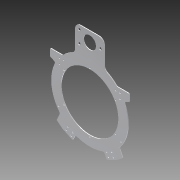
# Autodesk Inventor part: Tower_Top
Saved by Autodesk Inventor 2014 SP1 (Build 180222100, 222)
## iProperties
Created: 2012-02-04
Part Number: Tower_Top
Material: Aluminum-6061
Document SubType Name: Modeling
Designer: eagecat
Density: 2.71 g/cm^3
Mass: 552.559 g
Surface Area: 1384.69 cm^2
Volume: 203.896 cm^3
Appearance: Aluminum - Polished
Author: eagecat
Autodesk Inventor part; units mm, degrees
ref_plane "YZ Plane" through (0, 0, 0) normal (1, 0, 0) x (0, 1, 0)
ref_plane "XZ Plane" through (0, 0, 0) normal (0, 1, 0) x (-1, 0, 0)
ref_plane "XY Plane" through (0, 0, 0) normal (0, 0, 1) x (1, 0, 0)
sketch "Sketch1" plane through (0, 0, 0) normal (0, 0, 1) x (1, 0, 0)
  circle A0 centre (0, 0) radius 177.8
  circle A1 centre (0, 0) radius 132.461
  circle A2 centre (0, 0) radius 137.541 construction
  circle A3 centre (0, 137.541) radius 3.3782
  circle A4 centre (-119.114, 68.7705) radius 3.3782
  circle A5 centre (-119.114, -68.7705) radius 3.3782
  circle A6 centre (0, -137.541) radius 3.3782
  circle A7 centre (119.114, -68.7705) radius 3.3782
  circle A8 centre (119.114, 68.7705) radius 3.3782
  dimension "d2" = 275.082
  dimension "d0" = 355.6
  dimension "d1" = 264.922
  dimension "d3" = 6.7564
  dimension "d6" = 360
  constraints: 8 centre point, 3 coincident, 1 vertical alignment, 15 other
  measures "d0" diameter of A0
  measures "d1" diameter of A1
  measures "d3" diameter of A3
extrude "Extrusion1" add sketch "Sketch1" along normal blind 3.175
sketch "Sketch2" plane through (0, 0, 0) normal (0, 0, 1) x (1, 0, 0)
  line L0 (177.8, 120.269) -> (152.4, 120.269) construction
  line L1 (152.4, 120.269) -> (152.4, 94.869) construction
  line L2 (152.4, 94.869) -> (177.8, 94.869) construction
  line L3 (177.8, 94.869) -> (177.8, 120.269) construction
  line L4 (-176.2125, 96.4565) -> (-176.2125, 118.6815) construction
  line L5 (-176.2125, 118.6815) -> (-153.9875, 118.6815) construction
  line L6 (-153.9875, 118.6815) -> (-153.9875, 96.4565) construction
  line L7 (-153.9875, 96.4565) -> (-176.2125, 96.4565) construction
  line L8 (-177.8, 120.269) -> (-152.4, 120.269) construction
  line L9 (-177.8, 94.869) -> (-177.8, 120.269) construction
  line L10 (-152.4, 94.869) -> (-177.8, 94.869) construction
  line L11 (-152.4, 120.269) -> (-152.4, 94.869) construction
  line L12 (-131.8407, -121.2351) -> (-142.3056, -143.6999) construction
  line L13 (-111.6944, -130.6201) -> (-131.8407, -121.2351) construction
  line L14 (-122.1593, -153.0849) -> (-111.6944, -130.6201) construction
  line L15 (-142.3056, -143.6999) -> (-122.1593, -153.0849) construction
  line L16 (-144.4922, -144.6342) -> (-132.5322, -118.9602) construction
  line L17 (-121.4678, -155.3598) -> (-144.4922, -144.6342) construction
  line L18 (-109.5078, -129.6858) -> (-121.4678, -155.3598) construction
  line L19 (-132.5322, -118.9602) -> (-109.5078, -129.6858) construction
  line L20 (-108.1537, -135.5008) -> (-124.2421, -170.0373) construction
  line L21 (-81.532, -189.9334) -> (-124.2421, -170.0373) construction
  line L22 (-63.9062, -159.6156) -> (-77.3132, -188.396) construction
  line L23 (-108.1537, -135.5008) -> (-65.4435, -155.3968) construction
  circle A0 centre (109.1684, -166.5516) radius 3.3782 construction
  circle A1 centre (86.144, -177.2772) radius 3.3782 construction
  circle A2 centre (101.1241, -149.2833) radius 3.3782 construction
  circle A3 centre (78.0998, -160.0089) radius 3.3782 construction
  line L24 (108.1537, -135.5009) -> (124.2422, -170.0374) construction
  line L25 (108.1537, -135.5009) -> (62.5655, -156.7376) construction
  line L26 (62.5655, -156.7376) -> (78.6539, -191.2742) construction
  line L27 (78.6539, -191.2742) -> (124.2422, -170.0374) construction
  line L28 (142.3056, -143.6999) -> (131.8407, -121.2351) construction
  line L29 (122.1593, -153.0849) -> (142.3056, -143.6999) construction
  line L30 (111.6944, -130.6201) -> (122.1593, -153.0849) construction
  line L31 (131.8407, -121.2351) -> (111.6944, -130.6201) construction
  line L32 (132.5322, -118.9602) -> (144.4922, -144.6342) construction
  line L33 (109.5078, -129.6858) -> (132.5322, -118.9602) construction
  line L34 (121.4678, -155.3598) -> (109.5078, -129.6858) construction
  line L35 (144.4922, -144.6342) -> (121.4678, -155.3598) construction
  line L36 (0, 251.6148) -> (0, -265.089) construction
  line L37 (-256.032, 0) -> (256.032, 0) construction
  circle A4 centre (0, 0) radius 132.461 construction
  circle A5 centre (119.114, 68.7705) radius 3.3782 construction
  circle A6 centre (119.114, -68.7705) radius 3.3782 construction
  circle A7 centre (0, -137.541) radius 3.3782 construction
  circle A8 centre (-119.114, -68.7705) radius 3.3782 construction
  circle A9 centre (-119.114, 68.7705) radius 3.3782 construction
  circle A10 centre (0, 137.541) radius 3.3782 construction
  circle A11 centre (0, 0) radius 177.8 construction
  line L38 (-152.9297, -147.7089) -> (-124.2421, -170.0373)
  line L39 (-78.6539, -191.2741) -> (-124.2421, -170.0373)
  arc A12 (-58.5237, -167.8923) -> (-70.1072, -172.927) centre (-61.473, -176.9492) ccw
  line L40 (-70.1072, -172.927) -> (-78.6539, -191.2741)
  arc A13 (-138.5859, -111.3858) -> (-58.5237, -167.8923) centre (0, 0) ccw
  line L41 (-152.9297, -147.7089) -> (-139.107, -118.0362)
  arc A14 (-139.107, -118.0362) -> (-138.5859, -111.3858) centre (-147.7411, -114.0141) ccw
  line L42 (131.8407, -121.2351) -> (142.3056, -143.6999) construction
  line L43 (111.6944, -130.6201) -> (131.8407, -121.2351) construction
  line L44 (122.1593, -153.0849) -> (111.6944, -130.6201) construction
  line L45 (142.3056, -143.6999) -> (122.1593, -153.0849) construction
  line L46 (144.4922, -144.6342) -> (132.5322, -118.9602) construction
  line L47 (121.4678, -155.3598) -> (144.4922, -144.6342) construction
  line L48 (109.5078, -129.6858) -> (121.4678, -155.3598) construction
  line L49 (132.5322, -118.9602) -> (109.5078, -129.6858) construction
  circle A15 centre (109.1684, -166.5516) radius 3.3782 construction
  circle A16 centre (86.144, -177.2772) radius 3.3782 construction
  circle A17 centre (101.1241, -149.2833) radius 3.3782 construction
  circle A18 centre (78.0998, -160.0089) radius 3.3782 construction
  line L50 (108.1537, -135.5009) -> (124.2422, -170.0374) construction
  line L51 (78.6539, -191.2742) -> (124.2422, -170.0374) construction
  line L52 (62.5655, -156.7376) -> (78.6539, -191.2742) construction
  line L53 (108.1537, -135.5009) -> (62.5655, -156.7376) construction
  line L54 (152.9297, -147.7089) -> (124.2422, -170.0374)
  line L55 (78.6539, -191.2742) -> (124.2422, -170.0374)
  arc A19 (70.1072, -172.927) -> (58.5237, -167.8923) centre (61.473, -176.9492) ccw
  line L56 (70.1072, -172.927) -> (78.6539, -191.2742)
  arc A20 (58.5237, -167.8923) -> (138.5859, -111.3858) centre (0, 0) ccw
  line L57 (152.9297, -147.7089) -> (139.107, -118.0362)
  arc A21 (138.5859, -111.3858) -> (139.107, -118.0362) centre (147.7411, -114.0141) ccw
  line L58 (-182.88, 91.694) -> (-164.4375, 83.1028)
  line L59 (-182.88, 125.349) -> (-128.7113, 125.349)
  line L60 (-182.88, 125.349) -> (-182.88, 91.694)
  arc A22 (-161.3561, 74.6795) -> (-164.4375, 83.1028) centre (-167.1189, 77.3467) ccw
  arc A23 (-128.7113, 125.349) -> (-124.273, 127.1577) centre (-128.7113, 131.699) ccw
  arc A24 (-124.273, 127.1577) -> (-161.3561, 74.6795) centre (0, 0) ccw
  line L61 (176.2125, 96.4565) -> (176.2125, 118.6815) construction
  line L62 (176.2125, 118.6815) -> (153.9875, 118.6815) construction
  line L63 (153.9875, 118.6815) -> (153.9875, 96.4565) construction
  line L64 (153.9875, 96.4565) -> (176.2125, 96.4565) construction
  line L65 (177.8, 120.269) -> (152.4, 120.269) construction
  line L66 (177.8, 94.869) -> (177.8, 120.269) construction
  line L67 (152.4, 94.869) -> (177.8, 94.869) construction
  line L68 (152.4, 120.269) -> (152.4, 94.869) construction
  circle A25 centre (119.114, 68.7705) radius 3.3782 construction
  line L69 (182.88, 91.694) -> (164.4375, 83.1028)
  line L70 (182.88, 125.349) -> (128.7113, 125.349)
  line L71 (182.88, 125.349) -> (182.88, 91.694)
  arc A26 (164.4375, 83.1028) -> (161.3561, 74.6795) centre (167.1189, 77.3467) ccw
  arc A27 (124.273, 127.1577) -> (128.7113, 125.349) centre (128.7113, 131.699) ccw
  arc A28 (161.3561, 74.6795) -> (124.273, 127.1577) centre (0, 0) ccw
  arc A29 (-108.9915, -163.1779) -> (-109.3417, -163.1777) centre (-109.1683, -166.5515) ccw projected
  arc A30 (-85.9671, -173.9036) -> (-86.3174, -173.9034) centre (-86.144, -177.2771) ccw projected
  arc A31 (-100.9473, -145.9097) -> (-101.2975, -145.9095) centre (-101.1241, -149.2832) ccw projected
  arc A32 (-77.9229, -156.6353) -> (-78.2732, -156.6351) centre (-78.0998, -160.0089) ccw projected
  line L72 (-83.178, -156.6326) -> (-78.2732, -156.6351) projected
  line L73 (-77.9229, -156.6353) -> (-73.2656, -156.6377) projected
  arc A33 (-73.0184, -163.3851) -> (-73.2656, -156.6377) centre (-73.0198, -160.0069) ccw projected
  line L74 (-73.0184, -163.3851) -> (-83.1784, -163.389) projected
  arc A34 (-83.178, -156.6326) -> (-83.1784, -163.389) centre (-83.1797, -160.0108) ccw projected
  line L75 (-114.2466, -163.1752) -> (-109.3417, -163.1777) projected
  line L76 (-108.9915, -163.1779) -> (-104.3342, -163.1803) projected
  arc A35 (-104.087, -169.9277) -> (-104.3342, -163.1803) centre (-104.0883, -166.5495) ccw projected
  line L77 (-104.087, -169.9277) -> (-114.247, -169.9316) projected
  arc A36 (-114.2466, -163.1752) -> (-114.247, -169.9316) centre (-114.2483, -166.5534) ccw projected
  line L78 (-106.2024, -145.907) -> (-101.2975, -145.9095) projected
  line L79 (-100.9473, -145.9097) -> (-96.29, -145.912) projected
  arc A37 (-96.0428, -152.6595) -> (-96.29, -145.912) centre (-96.0441, -149.2813) ccw projected
  line L80 (-96.0428, -152.6595) -> (-106.2028, -152.6634) projected
  arc A38 (-106.2024, -145.907) -> (-106.2028, -152.6634) centre (-106.2041, -149.2852) ccw projected
  line L81 (-85.9671, -173.9036) -> (-81.3098, -173.9059) projected
  arc A39 (-81.0627, -180.6534) -> (-81.3098, -173.9059) centre (-81.064, -177.2752) ccw projected
  line L82 (-81.0627, -180.6534) -> (-91.2227, -180.6573) projected
  arc A40 (-91.2223, -173.9009) -> (-91.2227, -180.6573) centre (-91.224, -177.2791) ccw projected
  line L83 (-91.2223, -173.9009) -> (-86.3174, -173.9034) projected
  arc A41 (-63.9062, -159.6156) -> (-65.4435, -155.3968) centre (-66.7842, -158.2749) ccw projected
  arc A42 (-81.532, -189.9334) -> (-77.3132, -188.396) centre (-80.1912, -187.0553) ccw projected
  dimension "d11" = 6.35
  dimension "d12" = 9.525
  dimension "d13" = 9.525
  dimension "d14" = 6.35
  dimension "d23" = 3.175
  dimension "d24" = 5.08
  dimension "d25" = 5.08
  dimension "d26" = 6.35
  dimension "d27" = 6.35
  constraints: 36 end point, 28 point on circle, 20 symmetric about line, 17 centre point, 8 tangent, 3 perpendicular, 2 concentric, 2 parallel, 2 point on line, 1 collinear, 11 other
  measures "d11" distance from line of L17 L38.start
  measures "d12" radius of A12
  measures "d13" radius of A14
  measures "d14" distance between parallel lines of L16 L41
  measures "d23" distance from line of L10 L58.start
  measures "d24" distance between parallel lines of L60 L9
  measures "d25" distance between parallel lines of L59 L8
  measures "d26" radius of A23
  measures "d27" radius of A22
extrude "Extrusion5" add sketch "Sketch2" along normal blind 3.175 contours L41 A14 A13 L78 A38 L80 A37 A34 L74 A33 A12 L40 A42 L39 L38 | A42 L40 L39 | A13 A37 L80 A38 L78 | A13 A33 L74 A34 | L54 L55 L56 A19 A20 A21 L57 | L60 L59 A23 A24 A22 L58 | L69 A26 A28 A27 L70 L71 | L76 A35 L77 A36 L75 A29 | L81 A39 L82 A40 L83 A30
sketch "Sketch3" plane through (0, 0, 0) normal (0, 0, 1) x (1, 0, 0)
  circle A0 centre (109.1684, -166.5516) radius 3.3782 construction
  circle A1 centre (86.144, -177.2772) radius 3.3782 construction
  circle A2 centre (101.1241, -149.2833) radius 3.3782 construction
  circle A3 centre (78.0998, -160.0089) radius 3.3782 construction
  line L0 (124.2422, -170.0374) -> (108.1537, -135.5009) construction
  line L1 (124.2422, -170.0374) -> (78.6539, -191.2742) construction
  line L2 (78.6539, -191.2742) -> (62.5655, -156.7376) construction
  line L3 (62.5655, -156.7376) -> (108.1537, -135.5009) construction
  line L4 (-124.2421, -170.0373) -> (-108.1537, -135.5008) construction
  line L5 (-65.4435, -155.3968) -> (-108.1537, -135.5008) construction
  line L6 (-77.3132, -188.396) -> (-63.9062, -159.6156) construction
  line L7 (-124.2421, -170.0373) -> (-81.532, -189.9334) construction
  circle A4 centre (-109.1684, -166.5516) radius 3.3782
  circle A5 centre (-86.144, -177.2772) radius 3.3782
  circle A6 centre (-78.0998, -160.0089) radius 3.3782
  circle A7 centre (-101.1241, -149.2833) radius 3.3782
  circle A8 centre (78.0998, -160.0089) radius 3.3782
  circle A9 centre (86.144, -177.2772) radius 3.3782
  circle A10 centre (109.1684, -166.5516) radius 3.3782
  circle A11 centre (101.1241, -149.2833) radius 3.3782
  arc A12 (-108.9915, -163.1779) -> (-109.3417, -163.1777) centre (-109.1683, -166.5515) ccw projected
  arc A13 (-85.9671, -173.9036) -> (-86.3174, -173.9034) centre (-86.144, -177.2771) ccw projected
  arc A14 (-100.9473, -145.9097) -> (-101.2975, -145.9095) centre (-101.1241, -149.2832) ccw projected
  arc A15 (-77.9229, -156.6353) -> (-78.2732, -156.6351) centre (-78.0998, -160.0089) ccw projected
  line L8 (-86.3174, -173.9034) -> (-91.2223, -173.9009) projected
  arc A16 (-91.2223, -173.9009) -> (-91.2227, -180.6573) centre (-91.224, -177.2791) ccw projected
  line L9 (-91.2227, -180.6573) -> (-81.0627, -180.6534) projected
  arc A17 (-81.0627, -180.6534) -> (-81.3098, -173.9059) centre (-81.064, -177.2752) ccw projected
  line L10 (-81.3098, -173.9059) -> (-85.9671, -173.9036) projected
  line L11 (-101.2975, -145.9095) -> (-106.2024, -145.907) projected
  arc A18 (-106.2024, -145.907) -> (-106.2028, -152.6634) centre (-106.2041, -149.2852) ccw projected
  line L12 (-106.2028, -152.6634) -> (-96.0428, -152.6595) projected
  arc A19 (-96.0428, -152.6595) -> (-96.29, -145.912) centre (-96.0441, -149.2813) ccw projected
  line L13 (-96.29, -145.912) -> (-100.9473, -145.9097) projected
  line L14 (-109.3417, -163.1777) -> (-114.2466, -163.1752) projected
  arc A20 (-114.2466, -163.1752) -> (-114.247, -169.9316) centre (-114.2483, -166.5534) ccw projected
  line L15 (-114.247, -169.9316) -> (-104.087, -169.9277) projected
  arc A21 (-104.087, -169.9277) -> (-104.3342, -163.1803) centre (-104.0883, -166.5495) ccw projected
  line L16 (-104.3342, -163.1803) -> (-108.9915, -163.1779) projected
  line L17 (-78.2732, -156.6351) -> (-83.178, -156.6326) projected
  arc A22 (-83.178, -156.6326) -> (-83.1784, -163.389) centre (-83.1797, -160.0108) ccw projected
  line L18 (-83.1784, -163.389) -> (-73.0184, -163.3851) projected
  arc A23 (-73.0184, -163.3851) -> (-73.2656, -156.6377) centre (-73.0198, -160.0069) ccw projected
  line L19 (-73.2656, -156.6377) -> (-77.9229, -156.6353) projected
  arc A24 (-63.9062, -159.6156) -> (-65.4435, -155.3968) centre (-66.7842, -158.2749) ccw projected
  arc A25 (-81.532, -189.9334) -> (-77.3132, -188.396) centre (-80.1912, -187.0553) ccw projected
  point P0 (0, 0)
  constraints: 8 centre point, 8 equal radius, 4 coincident
extrude "Extrusion4" cut sketch "Sketch3" along normal blind 127 contours A4 | A5 | A6 | A7 | A8 | A9 | A10 | A11
fillet "Fillet1" radius 3.175 1 edges at (-182.88, 125.349, 1.5875)
fillet "Fillet2" radius 3.175 1 edges at (-182.88, 91.694, 1.5875)
fillet "Fillet3" radius 3.175 8 edges at (182.88, 125.349, 1.5875) (182.88, 91.694, 1.5875) (152.9297, -147.7089, 1.5875) (124.2422, -170.0374, 1.5875) (78.6539, -191.2742, 1.5875) (-78.6539, -191.2741, 1.5875) (-124.2421, -170.0373, 1.5875) (-152.9297, -147.7089, 1.5875)
sketch "Sketch4" plane through (0, 0, 0) normal (0, 0, -1) x (-1, 0, 0)
  arc A0 (130.175, 72.644) -> (133.35, 69.469) centre (133.35, 72.644) ccw construction
  line L0 (146.05, 69.469) -> (133.35, 69.469) construction
  arc A1 (146.05, 69.469) -> (149.225, 72.644) centre (146.05, 72.644) ccw construction
  line L1 (149.225, 85.344) -> (149.225, 72.644) construction
  line L2 (149.225, 85.344) -> (147.1295, 85.344) construction
  line L3 (147.1295, 85.344) -> (147.1295, 88.519) construction
  line L4 (147.1295, 88.519) -> (148.717, 88.519) construction
  line L5 (148.717, 88.519) -> (148.717, 120.269) construction
  line L6 (114.3, 120.269) -> (148.717, 120.269) construction
  arc A2 (114.3, 120.269) -> (111.125, 117.094) centre (114.3, 117.094) ccw construction
  line L7 (111.125, 98.044) -> (111.125, 117.094) construction
  arc A3 (111.125, 98.044) -> (114.3, 94.869) centre (114.3, 98.044) ccw construction
  line L8 (114.3, 94.869) -> (127, 94.869) construction
  arc A4 (130.175, 91.694) -> (127, 94.869) centre (127, 91.694) ccw construction
  line L9 (130.175, 91.694) -> (130.175, 72.644) construction
  arc A5 (136.3218, 77.089) -> (143.0782, 77.089) centre (139.7, 77.089) ccw construction
  line L10 (136.3218, 77.089) -> (136.3218, 87.249) construction
  arc A6 (143.0782, 87.249) -> (136.3218, 87.249) centre (139.7, 87.249) ccw construction
  line L11 (143.0782, 87.249) -> (143.0782, 77.089) construction
  line L12 (143.0782, 112.649) -> (143.0782, 102.489) construction
  arc A7 (136.3218, 102.489) -> (143.0782, 102.489) centre (139.7, 102.489) ccw construction
  line L13 (136.3218, 102.489) -> (136.3218, 112.649) construction
  arc A8 (143.0782, 112.649) -> (136.3218, 112.649) centre (139.7, 112.649) ccw construction
  line L14 (124.0282, 112.649) -> (124.0282, 102.489) construction
  arc A9 (117.2718, 102.489) -> (124.0282, 102.489) centre (120.65, 102.489) ccw construction
  line L15 (117.2718, 102.489) -> (117.2718, 112.649) construction
  arc A10 (124.0282, 112.649) -> (117.2718, 112.649) centre (120.65, 112.649) ccw construction
  arc A11 (-133.35, 69.469) -> (-130.175, 72.644) centre (-133.35, 72.644) ccw construction
  line L16 (-130.175, 91.694) -> (-130.175, 72.644) construction
  arc A12 (-127, 94.869) -> (-130.175, 91.694) centre (-127, 91.694) ccw construction
  line L17 (-114.3, 94.869) -> (-127, 94.869) construction
  arc A13 (-114.3, 94.869) -> (-111.125, 98.044) centre (-114.3, 98.044) ccw construction
  line L18 (-111.125, 98.044) -> (-111.125, 117.094) construction
  arc A14 (-111.125, 117.094) -> (-114.3, 120.269) centre (-114.3, 117.094) ccw construction
  line L19 (-114.3, 120.269) -> (-148.717, 120.269) construction
  line L20 (-148.717, 88.519) -> (-148.717, 120.269) construction
  line L21 (-147.1295, 88.519) -> (-148.717, 88.519) construction
  line L22 (-147.1295, 85.344) -> (-147.1295, 88.519) construction
  line L23 (-149.225, 85.344) -> (-147.1295, 85.344) construction
  line L24 (-149.225, 85.344) -> (-149.225, 72.644) construction
  arc A15 (-149.225, 72.644) -> (-146.05, 69.469) centre (-146.05, 72.644) ccw construction
  line L25 (-146.05, 69.469) -> (-133.35, 69.469) construction
  arc A16 (-143.0782, 77.089) -> (-136.3218, 77.089) centre (-139.7, 77.089) ccw construction
  line L26 (-143.0782, 87.249) -> (-143.0782, 77.089) construction
  arc A17 (-136.3218, 87.249) -> (-143.0782, 87.249) centre (-139.7, 87.249) ccw construction
  line L27 (-136.3218, 77.089) -> (-136.3218, 87.249) construction
  line L28 (-143.0782, 112.649) -> (-143.0782, 102.489) construction
  arc A18 (-136.3218, 112.649) -> (-143.0782, 112.649) centre (-139.7, 112.649) ccw construction
  line L29 (-136.3218, 102.489) -> (-136.3218, 112.649) construction
  arc A19 (-143.0782, 102.489) -> (-136.3218, 102.489) centre (-139.7, 102.489) ccw construction
  line L30 (-124.0282, 112.649) -> (-124.0282, 102.489) construction
  arc A20 (-117.2718, 112.649) -> (-124.0282, 112.649) centre (-120.65, 112.649) ccw construction
  line L31 (-117.2718, 102.489) -> (-117.2718, 112.649) construction
  arc A21 (-124.0282, 102.489) -> (-117.2718, 102.489) centre (-120.65, 102.489) ccw construction
  line L32 (120.65, 112.649) -> (120.65, 102.489) construction
  line L33 (139.7, 112.649) -> (139.7, 102.489) construction
  line L34 (139.7, 87.249) -> (139.7, 77.089) construction
  circle A22 centre (120.65, 107.569) radius 3.3782
  circle A23 centre (139.7, 107.569) radius 3.3782
  circle A24 centre (139.7, 82.169) radius 3.3782
  line L35 (-139.7, 112.649) -> (-139.7, 102.489) construction
  line L36 (-120.65, 112.649) -> (-120.65, 102.489) construction
  line L37 (-139.7, 87.249) -> (-139.7, 77.089) construction
  circle A25 centre (-139.7, 107.569) radius 3.3782
  circle A26 centre (-120.65, 107.569) radius 3.3782
  circle A27 centre (-139.7, 82.169) radius 3.3782
  constraints: 12 end point, 6 centre point, 6 equal length, 6 midpoint, 4 tangent
extrude "Extrusion6" cut sketch "Sketch4" against normal blind 25.4
sketch "Sketch6" plane through (0, 0, 3.175) normal (0, 0, 1) x (1, 0, 0)
  arc A0 (138.5859, -111.3858) -> (161.3561, 74.6795) centre (0, 0) ccw construction
  arc A1 (138.5859, -111.3858) -> (161.3561, 74.6795) centre (0, 0) ccw construction
  circle A2 centre (-48.7258, 267.14) radius 2.5 construction
  circle A3 centre (-48.7258, 267.14) radius 5.95 construction
  circle A4 centre (48.7258, 238.76) radius 2.5 construction
  circle A5 centre (48.7258, 238.76) radius 5.95 construction
  circle A6 centre (-48.7258, 210.38) radius 2.5 construction
  circle A7 centre (-48.7258, 210.38) radius 5.95 construction
  circle A8 centre (48.7258, 238.76) radius 7.1 construction
  circle A9 centre (-48.7258, 267.14) radius 7.1 construction
  circle A10 centre (-48.7258, 210.38) radius 7.1 construction
  line L0 (-42.3758, 286.19) -> (42.3758, 286.19)
  arc A11 (-42.3758, 286.19) -> (-67.7758, 260.79) centre (-42.3758, 260.79) ccw
  arc A12 (67.7758, 260.79) -> (42.3758, 286.19) centre (42.3758, 260.79) ccw
  line L1 (-67.7758, 260.79) -> (-67.7758, 180.5783)
  line L2 (67.7758, 260.79) -> (67.7758, 180.5783)
  arc A13 (-81.5289, 158.006) -> (-67.7758, 180.5783) centre (-93.1758, 180.5783) ccw
  arc A14 (67.7758, 180.5783) -> (81.5289, 158.006) centre (93.1758, 180.5783) ccw
  circle A15 centre (-48.7258, 267.14) radius 6.223
  circle A16 centre (48.7258, 238.76) radius 6.223
  circle A17 centre (-48.7258, 210.38) radius 6.223
  arc A18 (81.5289, 158.006) -> (-81.5289, 158.006) centre (0, 0) ccw
  circle A19 centre (0, 238.76) radius 29.21
  point P0 (124.273, 127.1577)
  point P1 (25.4, 175.9764)
  point P2 (-25.4, 175.9764)
  point P3 (-124.273, 127.1577)
  dimension "d50" = 25.4
  dimension "d51" = 25.4
  dimension "d52" = 19.05
  dimension "d53" = 19.05
  dimension "d54" = 19.05
  dimension "d55" = 25.4
  dimension "d56" = 12.446
  dimension "d57" = 12.446
  dimension "d58" = 12.446
  dimension "d63" = 58.42
  constraints: 12 point on circle, 9 centre point, 8 tangent, 6 end point, 4 coincident, 2 equal radius, 1 horizontal, 1 parallel, 1 perpendicular, 1 other
  measures "d50" radius of A11
  measures "d51" radius of A13
  measures "d52" distance from line of L1 A3.centre
  measures "d53" distance from line of L0 A2.centre
  measures "d54" distance from line of L2 A8.centre
  measures "d55" radius of A14
  measures "d56" diameter of A15
  measures "d57" diameter of A16
  measures "d58" diameter of A17
  measures "d63" diameter of A19
extrude "Extrusion10" add sketch "Sketch6" against normal blind 3.175
sketch "Sketch7" plane through (0, 0, 0) normal (0, 0, -1) x (-1, 0, 0)
  circle A0 centre (-143.8474, -86.121) radius 3.3782 projected
  circle A1 centre (143.8474, -86.121) radius 3.3782 projected
  point P0 (245.6114, -73.0705)
  constraints: 1 other
extrude "Extrusion11" cut sketch "Sketch7" against normal blind 25.4
equation "\"d57\" = d56"
equation "\"d58\" = d56"
body "Solid1"
